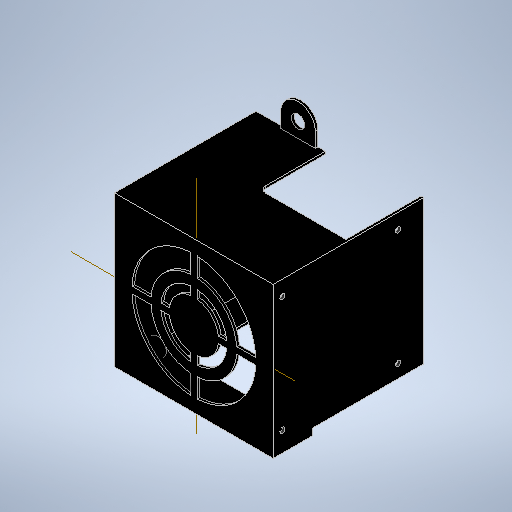
# Autodesk Inventor part: Fan Cover
Saved by Autodesk Inventor 2025.2 (Build 292293000, 293)
## iProperties
Manager: J. Wilburn
Created: 2025-03-12
Part Number: Fan Cover
Material: Aluminum 6061
Document SubType Name: Modeling
Designer: MAL16204
Density: 2.7 g/cm^3
Appearance: Anodized - Black
Mass: 17.0217 g
Surface Area: 161.072 cm^2
Volume: 6.30433 cm^3
Author: Richard Malstrom
Title: Fan Cover
Subject: Ender 3 Pro Assembly
Autodesk Inventor part; units mm, degrees
ref_plane "YZ Plane" through (0, 0, 0) normal (1, 0, 0) x (0, 1, 0)
ref_plane "XZ Plane" through (0, 0, 0) normal (0, 1, 0) x (-1, 0, 0)
ref_plane "XY Plane" through (0, 0, 0) normal (0, 0, 1) x (1, 0, 0)
sketch "Sketch1" plane through (0, 0, 0) normal (0, 0, 1) x (1, 0, 0)
  line L0 (-24, 22.8) -> (24, 22.8)
  line L1 (24, 22.8) -> (24, -22.8)
  line L2 (24, -22.8) -> (-24, -22.8)
  line L3 (-24, -22.8) -> (-24, 22.8)
  circle A0 centre (-16, 16.05) radius 2.7
  circle A1 centre (16, 16.05) radius 2.7
  circle A2 centre (16, -15.95) radius 2.7
  circle A3 centre (-16, -15.95) radius 2.7
  line L4 (0, -31.92) -> (0, 31.92) projected
  line L5 (-33.6, 0) -> (33.6, 0) projected
  arc A4 (18.7233, 1) -> (1, 18.7233) centre (0, 0) ccw
  arc A5 (-1, 18.7233) -> (-18.7233, 1) centre (0, 0) ccw
  arc A6 (12.9615, 1) -> (1, 12.9615) centre (0, 0) ccw
  arc A7 (-1, 12.9615) -> (-12.9615, 1) centre (0, 0) ccw
  arc A8 (9.933, 1) -> (1, 9.933) centre (0, 0) ccw
  arc A9 (-1, 9.933) -> (-9.933, 1) centre (0, 0) ccw
  arc A10 (-9.9499, -1) -> (-1, -9.9499) centre (0, 0) ccw
  arc A11 (1, -9.933) -> (9.933, -1) centre (0, 0) ccw
  arc A12 (-12.9615, -1) -> (-1, -12.9615) centre (0, 0) ccw
  arc A13 (1, -12.9615) -> (12.9615, -1) centre (0, 0) ccw
  line L6 (-1, -18.7233) -> (-1, -12.9615)
  line L7 (-1, -9.9499) -> (-1, -7.4499)
  line L8 (1, -7.433) -> (1, -9.933)
  line L9 (1, -12.9615) -> (1, -18.7233)
  line L10 (-7.433, 1) -> (-9.933, 1)
  line L11 (-12.9615, 1) -> (-18.7233, 1)
  line L12 (-1, 7.433) -> (-1, 9.933)
  line L13 (-1, 12.9615) -> (-1, 18.7233)
  line L14 (1, 18.7233) -> (1, 12.9615)
  line L15 (1, 9.933) -> (1, 7.433)
  line L16 (18.7233, 1) -> (12.9615, 1)
  line L17 (9.933, 1) -> (7.433, 1)
  line L18 (7.433, -1) -> (9.933, -1)
  line L19 (12.9615, -1) -> (18.7233, -1)
  line L20 (-18.7233, -1) -> (-12.9615, -1)
  line L21 (-9.9499, -1) -> (-7.4499, -1)
  arc A14 (-7.4499, -1) -> (-1, -7.4499) centre (0, 0) ccw
  arc A15 (1, -7.433) -> (7.433, -1) centre (0, 0) ccw
  arc A16 (-1, 7.433) -> (-7.433, 1) centre (0, 0) ccw
  arc A17 (7.433, 1) -> (1, 7.433) centre (0, 0) ccw
  arc A18 (-18.7233, -1) -> (-0.9363, -18.7266) centre (0, 0) ccw
  arc A19 (0.9363, -18.7266) -> (18.7233, -1) centre (0, 0) ccw
  circle A20 centre (16, 16.05) radius 1
  circle A21 centre (-16, 16.05) radius 1
  circle A22 centre (-16, -15.95) radius 1
  circle A23 centre (16, -15.95) radius 1
  point P0 (-24, 0)
  point P1 (-24, 0)
  point P2 (0, 22.8)
  point P3 (0, 22.8)
  dimension "d4" = 48
  dimension "d5" = 45.6
  dimension "d6" = 5.4
  dimension "d7" = 5.4
  dimension "d8" = 5.4
  dimension "d9" = 5.4
  dimension "d10" = 16
  dimension "d11" = 16
  dimension "d12" = 15.95
  dimension "d13" = 16.05
  dimension "d22" = 2.5
  dimension "d28" = 2
  dimension "d29" = 2
  dimension "d30" = 2
  dimension "d31" = 2
  constraints: 40 end point, 34 parallel, 34 point on circle, 24 centre point, 7 coincident, 7 equal length, 6 midpoint, 5 horizontal, 3 horizontal alignment, 3 vertical alignment, 2 point on line, 1 perpendicular
  measures "d4" distance between parallel lines of L1 L3
  measures "d5" distance between parallel lines of L2 L0
  measures "d6" diameter of A0
  measures "d7" diameter of A1
  measures "d8" diameter of A2
  measures "d9" diameter of A3
  measures "d10" distance from line of L4 A3.centre
  measures "d11" distance from line of A2.centre L4
  measures "d12" distance from line of L5 A2.centre
  measures "d13" distance from line of L5 A1.centre
  measures "d22" distance of L10.start L10.end
  measures "d28" diameter of A20
  measures "d29" diameter of A21
  measures "d30" diameter of A22
  measures "d31" diameter of A23
extrude "Extrusion1" add sketch "Sketch1" along normal blind 0.8 contours L0 L4 L5 L3 | L0 L1 L5 L4 | L5 L4 L2 L3 | L5 L1 L2 L4 | A0 | A1 | A2 | A3 | A20 | A21 | A22 | A23
sketch "Sketch2" plane through (0, 0, 0) normal (0, 0, -1) x (-1, 0, 0)
  line L0 (-24, 22.8) -> (24, 22.8) projected
  line L1 (-24, -22.8) -> (-24, 22.8) projected
  line L2 (24, -22.8) -> (-24, -22.8) projected
  line L3 (24, 22.8) -> (24, -22.8) projected
  line L4 (23.2, 22) -> (-23.2, 22)
  line L5 (-23.2, 22) -> (-23.2, -22)
  line L6 (-23.2, -22) -> (23.2, -22)
  line L7 (23.2, -22) -> (23.2, 22)
  point P0 (0, 0)
  dimension "d25" = 0.8
  constraints: 8 end point, 3 other
  measures "d25" distance between parallel lines of L0 L4
extrude "Extrusion2" add sketch "Sketch2" along normal blind 42
sketch "Sketch3" plane through (0, 0, 0) normal (0, 0, -1) x (-1, 0, 0)
  circle A0 centre (-16, 16.05) radius 2.7
  circle A1 centre (16, 16.05) radius 2.7
  circle A2 centre (16, -15.95) radius 2.7
  circle A3 centre (-16, -15.95) radius 2.7
  line L0 (33.6, 0) -> (-33.6, 0) projected
  line L1 (0, -31.92) -> (0, 31.92) projected
  point P0 (0, 0)
  dimension "d32" = 5.4
  dimension "d33" = 5.4
  dimension "d34" = 5.4
  dimension "d35" = 5.4
  dimension "d36" = 16.05
  dimension "d37" = 15.95
  dimension "d38" = 16
  dimension "d39" = 16
  constraints: 4 centre point, 2 horizontal alignment, 2 vertical alignment
  measures "d32" diameter of A0
  measures "d33" diameter of A1
  measures "d34" diameter of A2
  measures "d35" diameter of A3
  measures "d36" distance from line of A1.centre L0
  measures "d37" distance from line of A2.centre L0
  measures "d38" distance from line of A3.centre L1
  measures "d39" distance from line of A2.centre L1
extrude "Extrusion3" add sketch "Sketch3" along normal blind 4.2
sketch "Sketch4" plane through (16, 16.05, -4.2) normal (0, 0, -1) x (-1, 0, 0)
  circle A0 centre (0, 0) radius 2.7 projected
  circle A1 centre (32, 0) radius 2.7 projected
  circle A2 centre (32, -32) radius 2.7 projected
  circle A3 centre (0, -32) radius 2.7 projected
  point P0 (16, -16.05)
  constraints: 4 coincident
hole "Hole1" at (16, 16.05, -4.2) at (-16, 16.05, -4.2) at (-16, -15.95, -4.2) at (16, -15.95, -4.2) direction (0, 0, 1) diameter 2.459 depth 4 thread size "M3x0.5" class "6H" standard "ISO Metric profile"
sketch "Sketch5" plane through (-24, 22.8, 0.8) normal (0, 1, 0) x (1, 0, 0)
  line L0 (0, 42.8) -> (48, 42.8) projected
  line L1 (48, 42.8) -> (21.8, 42.8)
  line L2 (0.8, 42.8) -> (47.2, 42.8) projected
  line L3 (47.2, 22.8) -> (21, 22.8)
  line L4 (21, 22.8) -> (21, 42.8)
  line L5 (21, 42.8) -> (47.2, 42.8)
  line L6 (47.2, 42.8) -> (47.2, 22.8)
  line L7 (48, 0) -> (48, 42.8) projected
  point P0 (24, 0.8)
  dimension "d53" = 26.2
  dimension "d54" = 20
  dimension "d55" = 0.8
  constraints: 10 end point, 2 horizontal, 2 parallel, 1 perpendicular, 1 point on line
  measures "d53" distance between parallel lines of L4 L6
  measures "d54" distance between parallel lines of L0 L3
  measures "d55" distance between parallel lines of L7 L6
extrude "Extrusion4" cut sketch "Sketch5" against normal up to surface (0.8 mm away)
sketch "Sketch6" plane through (-23.2, -22, 0) normal (0, 1, 0) x (1, 0, 0)
  line L0 (47.2, 42) -> (-0.8, 42) projected
  line L1 (46.4, 42) -> (8.2, 42)
  line L2 (8.2, 42) -> (8.2, 11)
  line L3 (8.2, 11) -> (46.4, 11)
  line L4 (46.4, 11) -> (46.4, 42)
  line L5 (47.2, 42) -> (47.2, -0.8) projected
  point P0 (23.2, 0)
  dimension "d56" = 0.8
  dimension "d57" = 38.2
  dimension "d58" = 31
  constraints: 8 end point, 2 parallel, 1 horizontal, 1 perpendicular, 1 point on line
  measures "d56" distance between parallel lines of L5 L4
  measures "d57" distance between parallel lines of L4 L2
  measures "d58" distance between parallel lines of L0 L3
extrude "Extrusion5" cut sketch "Sketch6" against normal up to surface (0.8 mm away)
fillet "Fillet1" radius 2 2 edges at (-3, 22.4, -22) (-15, -22.4, -11)
sketch "Sketch7" plane through (-24, -22.8, 0.8) normal (-1, 0, 0) x (0, 0, 1)
  line L0 (-38.3, 37.6) -> (-13.3, 37.6) construction
  line L1 (-38.3, 36.1) -> (-13.3, 36.1)
  line L2 (-13.3, 39.1) -> (-38.3, 39.1)
  arc A0 (-38.3, 39.1) -> (-38.3, 36.1) centre (-38.3, 37.6) ccw
  arc A1 (-13.3, 36.1) -> (-13.3, 39.1) centre (-13.3, 37.6) ccw
  line L3 (-42.8, 45.6) -> (0, 45.6) projected
  line L4 (-42.8, 0) -> (-42.8, 45.6) projected
  line L5 (-13.3, 34.1) -> (-38.3, 34.1)
  arc A2 (-38.3, 34.1) -> (-38.3, 31.1) centre (-38.3, 32.6) ccw
  line L6 (-38.3, 31.1) -> (-13.3, 31.1)
  arc A3 (-13.3, 31.1) -> (-13.3, 34.1) centre (-13.3, 32.6) ccw
  line L7 (-13.3, 29.1) -> (-38.3, 29.1)
  arc A4 (-38.3, 29.1) -> (-38.3, 26.1) centre (-38.3, 27.6) ccw
  line L8 (-38.3, 26.1) -> (-13.3, 26.1)
  arc A5 (-13.3, 26.1) -> (-13.3, 29.1) centre (-13.3, 27.6) ccw
  point P0 (-0.8, 22.8)
  point P1 (-25.8, 37.6)
  dimension "d63" = 3
  dimension "d64" = 25
  dimension "d65" = 8
  dimension "d66" = 17
  dimension "d69" = 5
  constraints: 16 end point, 12 point on circle, 6 centre point, 4 tangent, 1 horizontal, 1 midpoint, 1 parallel, 1 vertical, 20 other
  measures "d63" distance between parallel lines of L1 L2
  measures "d64" distance of L0.end L0.start
  measures "d65" distance from line of L3 point (-25.8, 37.6)
  measures "d66" distance from line of L4 point (-25.8, 37.6)
  measures "d69" distance of L2.start L5.start
extrude "Extrusion6" cut sketch "Sketch7" against normal up to surface (0.8 mm away)
sketch "Sketch8" plane through (24, -22.8, 0.8) normal (1, 0, 0) x (0, 0, -1)
  line L0 (0, 45.6) -> (42.8, 45.6) projected
  line L1 (42.8, 45.6) -> (42.8, 0) projected
  point P0 (0.8, 22.8)
  point P1 (2.8, 41)
  point P2 (37.8, 41)
  point P3 (37.8, 6)
  point P4 (2.8, 6)
  dimension "d76" = 4.6
  dimension "d77" = 39.6
  dimension "d78" = 40
  dimension "d79" = 5
  constraints: 2 horizontal alignment, 2 vertical alignment
  measures "d76" distance from line of L0 point (37.8, 41)
  measures "d77" distance from line of point (37.8, 6) L0
  measures "d78" distance from line of point (2.8, 6) L1
  measures "d79" distance from line of L1 point (37.8, 6)
hole "Hole2" at (24, 18.2, -2) at (24, 18.2, -37) at (24, -16.8, -37) at (24, -16.8, -2) direction (-1, 0, 0) diameter 1.567 depth 4.55 thread size "M2x0.4" class "6H" standard "ISO Metric profile"
sketch "Sketch9" plane through (0, 0, -42) normal (0, 0, -1) x (-1, 0, 0)
  line L0 (-24, -22.8) -> (-24, 22.8) projected
  line L1 (24, -22.8) -> (-24, -22.8) projected
  line L2 (-24, 22.8) -> (-23.2, 22.8)
  line L3 (-23.2, 22.8) -> (-23.2, -22.8)
  line L4 (-23.2, -22.8) -> (-24, -22.8)
  line L5 (-24, -22.8) -> (-24, 22.8)
  point P0 (0, 0)
  dimension "d87" = 0.8
  constraints: 8 end point, 2 parallel, 1 horizontal, 1 perpendicular, 1 point on line
  measures "d87" distance of L3.end L4.end
extrude "Extrusion7" add sketch "Sketch9" along normal blind 2.8
sketch "Sketch10" plane through (24, -22.8, 0.8) normal (1, 0, 0) x (0, 0, -1)
  line L0 (45.6, 0) -> (45.6, 45.6) projected
  line L1 (45.6, 0) -> (11.8, 0)
  line L2 (11.8, 0) -> (11.8, 2)
  line L3 (11.8, 2) -> (45.6, 2)
  line L4 (45.6, 2) -> (45.6, 0)
  point P0 (0.8, 22.8)
  point P1 (45.6, 2)
  dimension "d90" = 33.8
  dimension "d91" = 2
  constraints: 8 end point, 2 parallel, 1 horizontal, 1 perpendicular
  measures "d90" distance of L2.end L3.end
  measures "d91" distance of L1.end L2.end
extrude "Extrusion8" cut sketch "Sketch10" against normal up to surface (0.8 mm away)
sketch "Sketch11" plane through (0, 0, -42) normal (0, 0, -1) x (-1, 0, 0)
  circle A0 centre (10.5, 27.25) radius 2
  circle A1 centre (28, 8.35) radius 2
  line L0 (24, 22.8) -> (3, 22.8) projected
  arc A2 (15.75, 27.25) -> (5.25, 27.25) centre (10.5, 27.25) ccw
  line L1 (23.2, 22) -> (-23.2, 22) projected
  line L2 (5.25, 27.25) -> (5.25, 22.8)
  line L3 (15.75, 27.25) -> (15.75, 22.8)
  arc A3 (28, 4.35) -> (28, 12.35) centre (28, 8.35) ccw
  line L4 (28, 12.35) -> (24, 12.35)
  line L5 (24, 22.8) -> (24, -22.8) projected
  line L6 (28, 4.35) -> (24, 4.35)
  point P0 (0, 0)
  point P1 (10.5, 31.85)
  dimension "d94" = 4
  dimension "d95" = 4
  dimension "d96" = 28
  dimension "d97" = 27.25
  dimension "d98" = 10.5
  dimension "d99" = 8.35
  dimension "d100" = 31.85
  dimension "d101" = 8
  constraints: 8 end point, 5 tangent, 4 centre point, 4 point on circle, 3 perpendicular, 3 point on line, 2 coincident, 1 horizontal
  measures "d94" diameter of A0
  measures "d95" diameter of A1
  measures "d96" horizontal distance of point (0, 0) A1.centre
  measures "d97" vertical distance of A0.centre point (0, 0)
  measures "d98" horizontal distance of A0.centre point (0, 0)
  measures "d99" vertical distance of A1.centre point (0, 0)
  measures "d100" vertical distance of point (0, 0) point (10.5, 31.85)
  measures "d101" diameter of A3
extrude "Extrusion9" add sketch "Sketch11" against normal blind 0.8
body "Solid1"
